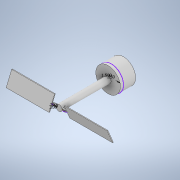
# Autodesk Inventor part: Main flyer
Saved by Autodesk Inventor 2021 (Build 250183000, 183)
## iProperties
Created: 2020-07-12
Part Number: Main flyer
Material: Generic
Document SubType Name: Modeling
Designer: saipr
Density: 1 g/cm^3
Appearance: Default
Author: saipr
Autodesk Inventor part; units mm, degrees
ref_plane "YZ Plane" through (0, 0, 0) normal (1, 0, 0) x (0, 1, 0)
ref_plane "XZ Plane" through (0, 0, 0) normal (0, 1, 0) x (-1, 0, 0)
ref_plane "XY Plane" through (0, 0, 0) normal (0, 0, 1) x (1, 0, 0)
sketch "Sketch1" plane through (0, 0, 0) normal (0, 0, 1) x (1, 0, 0)
  point P0 (0, 0)
sketch "Sketch2" plane through (0, 0, 0) normal (0, 0, 1) x (1, 0, 0)
  circle A0 centre (0, 0) radius 25.4
  dimension "d0" = 50.8
  constraints: 1 centre point, 1 coincident
  measures "d0" diameter of A0
extrude "Extrusion1" add sketch "Sketch2" along normal blind 6.35
sketch "Sketch3" plane through (0, 0, 6.35) normal (0, 0, 1) x (1, 0, 0)
  circle A0 centre (0, 0) radius 6.35
  dimension "d3" = 12.7
  constraints: 1 centre point, 1 coincident
  measures "d3" diameter of A0
extrude "Extrusion2" add sketch "Sketch3" along normal blind 101.6
sketch "Sketch4" plane through (0, 0, 107.95) normal (0, 0, 1) x (1, 0, 0)
  circle A0 centre (0, 0) radius 6.35 projected
  line L0 (-4.4901, 4.4901) -> (4.4901, 4.4901)
  line L1 (4.4901, 4.4901) -> (4.4901, -4.4901)
  line L2 (4.4901, -4.4901) -> (-4.4901, -4.4901)
  line L3 (-4.4901, -4.4901) -> (-4.4901, 4.4901)
  line L4 (-4.4901, 4.4901) -> (4.4901, -4.4901) construction
  line L5 (4.4901, 4.4901) -> (-4.4901, -4.4901) construction
  line L6 (-12.7, 1.905) -> (12.7, 1.905)
  line L7 (12.7, 1.905) -> (12.7, -1.905)
  line L8 (12.7, -1.905) -> (-12.7, -1.905)
  line L9 (-12.7, -1.905) -> (-12.7, 1.905)
  line L10 (-12.7, 1.905) -> (12.7, -1.905) construction
  line L11 (12.7, 1.905) -> (-12.7, -1.905) construction
  line L12 (-12.7, 0.7253) -> (-4.4901, 0.7253)
  line L13 (-4.4901, 0.7253) -> (-4.4901, -0.8127)
  line L14 (-4.4901, -0.8127) -> (-12.7, -0.8127)
  line L15 (-12.7, -0.8127) -> (-12.7, 0.7253)
  line L16 (12.7, 0.7253) -> (4.4901, 0.7253)
  line L17 (4.4901, 0.7253) -> (4.4901, -0.8127)
  line L18 (4.4901, -0.8127) -> (12.7, -0.8127)
  line L19 (12.7, -0.8127) -> (12.7, 0.7253)
  dimension "d7" = 25.4
  dimension "d8" = 3.81
  constraints: 40 end point, 8 parallel, 6 point on line, 4 horizontal, 4 midpoint, 4 perpendicular, 1 point on circle
  measures "d7" distance of L7.end L8.end
  measures "d8" distance of L6.end L7.end
extrude "Extrusion3" add sketch "Sketch4" against normal blind 3.175 contours L6 L7 L16 A0 | A0 L16 L1 L6 | L1 L8 L3 L6 | L6 L3 L12 A0 | A0 L12 L9 L6 | L18 A0 L8 L1 | L14 L3 L8 A0 | A0 L8 L9 L14 | L18 L7 L8 A0
sketch "Sketch5" plane through (6.0575, 1.905, 107.95) normal (0, 1, 0) x (1, 0, 0)
  line L0 (6.6425, 0) -> (0.2403, 0) projected
  line L1 (6.6425, 0) -> (-9.8567, 0)
  line L2 (6.6425, 0) -> (6.6425, 3.175) projected
  line L3 (6.6425, 0) -> (6.6425, 3.175)
  line L4 (0, 0) -> (0, 3.175) projected
  line L5 (6.6425, 3.175) -> (0, 3.175)
  line L6 (0, 3.175) -> (0, 0)
  line L7 (0, 0) -> (6.6425, 0)
  line L8 (-12.115, 3.175) -> (-12.3553, 3.175) projected
  line L9 (-18.7575, 0) -> (-12.115, 0)
  line L10 (-12.115, 0) -> (-12.115, 3.175)
  line L11 (-12.115, 3.175) -> (-18.7575, 3.175)
  line L12 (-18.7575, 3.175) -> (-18.7575, 0)
  line L13 (3.3212, 0) -> (3.3212, 3.175)
  circle A0 centre (3.3212, 1.5875) radius 1.5875
  line L14 (-18.7575, 0) -> (-12.366, 0) projected
  line L15 (-15.5617, 0) -> (-15.5617, 3.175)
  circle A1 centre (-15.5617, 1.5875) radius 1.5875
  point P0 (-6.0575, 107.95)
  constraints: 22 end point, 5 midpoint, 4 perpendicular, 2 collinear, 2 horizontal, 2 parallel, 2 vertical alignment, 1 point on line, 4 other
extrude "Extrusion4" add sketch "Sketch5" against normal blind 3.81 contours A0 L13 | L13 A0 | A1 L15 | L15 A1
ref_plane "Work Plane1" through (6.0575, 0, 107.95) normal (0, 1, 0) x (1, 0, 0)
sketch "Sketch6" plane through (6.0575, 0, 107.95) normal (0, 1, 0) x (1, 0, 0)
  line L0 (3.3212, 3.175) -> (0.2509, 3.175) projected
  line L1 (0.2509, 0) -> (3.3212, 0) projected
  line L2 (3.3212, 3.175) -> (3.3212, 0)
  circle A0 centre (3.3212, 1.5875) radius 1.651
  circle A1 centre (3.3212, 1.5875) radius 2.921
  line L3 (9.6712, 3.175) -> (9.6712, -0.0635)
  line L4 (9.6712, -0.0635) -> (3.3212, -0.0635)
  arc A2 (-15.5617, 0) -> (-15.5617, 3.175) centre (-15.5617, 1.5875) ccw projected
  circle A3 centre (-15.5617, 1.5875) radius 1.651
  circle A4 centre (-15.5617, 1.5875) radius 2.921
  line L5 (-15.5617, -0.0635) -> (-21.9117, -0.0635)
  line L6 (-21.9117, -0.0635) -> (-21.9117, 3.2385)
  line L7 (-21.9117, 3.2385) -> (-15.5617, 3.2385)
  line L8 (3.3212, 3.2385) -> (9.6712, 3.2385)
  line L9 (9.6712, 3.2385) -> (9.6712, 3.175)
  point P0 (-6.0575, 107.95)
  point P1 (5.7309, -0.0635)
  point P2 (5.7309, 3.2385)
  point P3 (-17.9714, -0.0635)
  point P4 (-17.9714, 3.2385)
  dimension "d19" = 3.302
  dimension "d20" = 5.842
  dimension "d22" = 6.35
  constraints: 16 end point, 4 centre point, 4 point on circle, 3 coincident, 3 perpendicular, 2 horizontal, 1 midpoint, 1 point on line, 1 vertical
  measures "d19" diameter of A3
  measures "d20" diameter of A4
  measures "d22" distance of L5.start L5.end
extrude "Extrusion5" add sketch "Sketch6" along normal mid plane 1.016 contours A0 L1 A1 L0 | L0 A1 L8 A0 | L8 A1 L4 A0 | A0 L4 A1 L1 | L8 L9 L3 L4 A1
extrude "Extrusion6" add sketch "Sketch6" along normal mid plane 1.016 contours A3 L7 A4 L5 | A3 L5 A4 L7 | A4 L5 L6 L7
sketch "Sketch7" plane through (-15.8542, -0.508, 108.0135) normal (-1, 0, 0) x (0, 0, 1)
  line L0 (0, 0) -> (0, 1.016) projected
  line L1 (0, 0.508) -> (-3.302, 0.508)
  line L2 (-3.302, 1.016) -> (-3.302, 0) projected
  line L3 (-3.2385, 2.413) -> (-0.0635, -1.397) construction
  line L4 (-0.0635, 2.413) -> (-3.2385, -1.397) construction
  line L5 (-3.2385, 2.413) -> (-1.651, -1.397)
  line L6 (-0.0635, -1.397) -> (-1.651, 2.413)
  line L7 (-1.651, -1.397) -> (3.2336, -13.1201)
  line L8 (3.2336, -13.1201) -> (4.8211, -13.1201)
  line L9 (4.8211, -13.1201) -> (-0.0635, -1.397)
  line L10 (-3.2385, 2.413) -> (-3.2385, 1.2333) projected
  line L11 (-3.2385, 2.413) -> (-8.1231, 14.1361)
  line L12 (-8.1231, 14.1361) -> (-6.5356, 14.1361)
  line L13 (-6.5356, 14.1361) -> (-1.651, 2.413)
  point P0 (-108.0135, 0.508)
  point P1 (-1.651, 0.508)
  dimension "d29" = 12.7
  dimension "d30" = 12.7
  constraints: 22 end point, 5 midpoint, 2 collinear, 2 parallel, 1 horizontal, 1 perpendicular
  measures "d29" distance of L8.end L3.end
  measures "d30" distance of L3.start L11.end
extrude "Extrusion8" add sketch "Sketch7" along normal blind 88.9
sketch "Sketch8" plane through (15.7288, -0.508, 104.7115) normal (1, 0, 0) x (0, 0, -1)
  line L0 (-3.302, 1.016) -> (-3.302, 0) projected
  line L1 (-3.302, 0.508) -> (-0.0635, 0.508)
  line L2 (-0.0635, 1.2333) -> (-0.0635, -0.3047) projected
  line L3 (-3.2385, 1.2333) -> (-3.2385, 2.413) projected
  line L4 (-0.0635, -1.397) -> (-3.2385, -1.397) projected
  line L5 (-1.651, 2.413) -> (-0.0635, 2.413)
  line L6 (-0.0635, 2.413) -> (-0.0635, -1.397)
  line L7 (-1.651, -1.397) -> (-3.2385, -1.397)
  line L8 (-3.2385, -1.397) -> (-3.2385, 2.413)
  line L9 (-3.2385, 2.413) -> (-0.0635, 2.413) projected
  line L10 (-3.2385, 2.413) -> (-1.651, -1.397)
  line L11 (-1.651, 2.413) -> (-0.0635, -1.397)
  line L12 (-1.651, -1.397) -> (3.2336, -13.1201)
  line L13 (3.2336, -13.1201) -> (4.8211, -13.1201)
  line L14 (4.8211, -13.1201) -> (-0.0635, -1.397)
  line L15 (-3.2385, 2.413) -> (-8.1231, 14.1361)
  line L16 (-8.1231, 14.1361) -> (-6.5356, 14.1361)
  line L17 (-6.5356, 14.1361) -> (-1.651, 2.413)
  point P0 (104.7115, 0.508)
  dimension "d31" = 12.7
  dimension "d32" = 12.7
  constraints: 26 end point, 5 parallel, 4 horizontal, 3 collinear, 1 midpoint, 1 perpendicular, 1 point on line
  measures "d31" distance of L7.start L12.end
  measures "d32" distance of L3.end L15.end
extrude "Extrusion9" add sketch "Sketch8" along normal blind 88.9 contours L10 L9 L11 L1 | L1 L11 L4 L10 | L15 L16 L17 L9 | L4 L14 L13 L12
sketch "Sketch9" plane through (0, 0, 0) normal (0, 0, -1) x (-1, 0, 0)
  circle A0 centre (0, 0) radius 25.4
  circle A1 centre (0, 0) radius 19.05
  circle A2 centre (0, 0) radius 3.175
  dimension "d35" = 38.1
  dimension "d38" = 6.35
  constraints: 3 centre point, 3 coincident
  measures "d35" diameter of A1
  measures "d38" diameter of A2
extrude "Extrusion10" add sketch "Sketch9" along normal blind 25.4 contours A0
extrude "Extrusion11" cut sketch "Sketch9" against normal blind 101.6 contours A2
body "Solid1"
